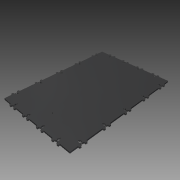
# Autodesk Inventor part: bottom
Saved by Autodesk Inventor 2014 (Build 180170000, 170)
## iProperties
Created: 2013-12-07
Part Number: bottom
Material: Plywood, Finish
Document SubType Name: Modeling
Designer: buben
Density: 0.552 g/cm^3
Appearance: Plywood - New
Author: buben
Subject: Laser Cutted
Autodesk Inventor part; units mm, degrees
ref_plane "YZ Plane" through (0, 0, 0) normal (1, 0, 0) x (0, 1, 0)
ref_plane "XZ Plane" through (0, 0, 0) normal (0, 1, 0) x (-1, 0, 0)
ref_plane "XY Plane" through (0, 0, 0) normal (0, 0, 1) x (1, 0, 0)
sketch "Sketch1" plane through (0, 0, 0) normal (0, 0, 1) x (1, 0, 0)
  line L0 (0, 0) -> (336, 0)
  line L1 (336, 0) -> (336, 489)
  line L2 (336, 489) -> (0, 489)
  line L3 (0, 489) -> (0, 0)
  dimension "d0" = 336
  dimension "d1" = 489
  constraints: 8 end point, 2 parallel, 1 horizontal, 1 perpendicular
  measures "d0" distance of L0.start L0.end
  measures "d1" distance of L2.end L0.start
extrude "Extrusion1" add sketch "Sketch1" along normal blind 6.5
sketch "Sketch6" plane through (0, 0, 6.5) normal (0, 0, 1) x (1, 0, 0)
  line L0 (0, 0) -> (336, 0) projected
  line L1 (336, 0) -> (336, 489) projected
  line L2 (336, 489) -> (0, 489) projected
  line L3 (0, 489) -> (0, 0) projected
  line L4 (54.75, 0) -> (59.25, 0)
  line L5 (59.25, 16.3) -> (54.75, 16.3)
  line L6 (61.75, 12.3) -> (61.75, 5)
  line L7 (52.25, 5) -> (52.25, 12.3)
  line L8 (54.75, 16.3) -> (54.75, 12.3)
  line L9 (54.75, 5) -> (54.75, 0)
  line L10 (59.25, 0) -> (59.25, 5)
  line L11 (59.25, 12.3) -> (59.25, 16.3)
  line L12 (61.75, 5) -> (59.25, 5)
  line L13 (54.75, 5) -> (52.25, 5)
  line L14 (52.25, 12.3) -> (54.75, 12.3)
  line L15 (59.25, 12.3) -> (61.75, 12.3)
  line L16 (128.75, 0) -> (133.25, 0)
  line L17 (133.25, 16.3) -> (128.75, 16.3)
  line L18 (135.75, 12.3) -> (135.75, 5)
  line L19 (126.25, 5) -> (126.25, 12.3)
  line L20 (128.75, 16.3) -> (128.75, 12.3)
  line L21 (128.75, 5) -> (128.75, 0)
  line L22 (133.25, 0) -> (133.25, 5)
  line L23 (133.25, 12.3) -> (133.25, 16.3)
  line L24 (135.75, 5) -> (133.25, 5)
  line L25 (128.75, 5) -> (126.25, 5)
  line L26 (126.25, 12.3) -> (128.75, 12.3)
  line L27 (133.25, 12.3) -> (135.75, 12.3)
  line L28 (202.75, 0) -> (207.25, 0)
  line L29 (207.25, 16.3) -> (202.75, 16.3)
  line L30 (209.75, 12.3) -> (209.75, 5)
  line L31 (200.25, 5) -> (200.25, 12.3)
  line L32 (202.75, 16.3) -> (202.75, 12.3)
  line L33 (202.75, 5) -> (202.75, 0)
  line L34 (207.25, 0) -> (207.25, 5)
  line L35 (207.25, 12.3) -> (207.25, 16.3)
  line L36 (209.75, 5) -> (207.25, 5)
  line L37 (202.75, 5) -> (200.25, 5)
  line L38 (200.25, 12.3) -> (202.75, 12.3)
  line L39 (207.25, 12.3) -> (209.75, 12.3)
  line L40 (276.75, 0) -> (281.25, 0)
  line L41 (281.25, 16.3) -> (276.75, 16.3)
  line L42 (283.75, 12.3) -> (283.75, 5)
  line L43 (274.25, 5) -> (274.25, 12.3)
  line L44 (276.75, 16.3) -> (276.75, 12.3)
  line L45 (276.75, 5) -> (276.75, 0)
  line L46 (281.25, 0) -> (281.25, 5)
  line L47 (281.25, 12.3) -> (281.25, 16.3)
  line L48 (283.75, 5) -> (281.25, 5)
  line L49 (276.75, 5) -> (274.25, 5)
  line L50 (274.25, 12.3) -> (276.75, 12.3)
  line L51 (281.25, 12.3) -> (283.75, 12.3)
  line L52 (0, 244.5) -> (336, 244.5) construction
  line L53 (54.75, 489) -> (59.25, 489)
  line L54 (59.25, 472.7) -> (54.75, 472.7)
  line L55 (61.75, 476.7) -> (61.75, 484)
  line L56 (52.25, 484) -> (52.25, 476.7)
  line L57 (54.75, 472.7) -> (54.75, 476.7)
  line L58 (54.75, 484) -> (54.75, 489)
  line L59 (59.25, 489) -> (59.25, 484)
  line L60 (59.25, 476.7) -> (59.25, 472.7)
  line L61 (61.75, 484) -> (59.25, 484)
  line L62 (54.75, 484) -> (52.25, 484)
  line L63 (52.25, 476.7) -> (54.75, 476.7)
  line L64 (59.25, 476.7) -> (61.75, 476.7)
  line L65 (128.75, 484) -> (126.25, 484)
  line L66 (135.75, 484) -> (133.25, 484)
  line L67 (128.75, 484) -> (128.75, 489)
  line L68 (128.75, 489) -> (133.25, 489)
  line L69 (133.25, 489) -> (133.25, 484)
  line L70 (126.25, 476.7) -> (128.75, 476.7)
  line L71 (126.25, 484) -> (126.25, 476.7)
  line L72 (133.25, 476.7) -> (135.75, 476.7)
  line L73 (135.75, 476.7) -> (135.75, 484)
  line L74 (128.75, 472.7) -> (128.75, 476.7)
  line L75 (133.25, 476.7) -> (133.25, 472.7)
  line L76 (133.25, 472.7) -> (128.75, 472.7)
  line L77 (202.75, 484) -> (200.25, 484)
  line L78 (209.75, 484) -> (207.25, 484)
  line L79 (202.75, 484) -> (202.75, 489)
  line L80 (202.75, 489) -> (207.25, 489)
  line L81 (207.25, 489) -> (207.25, 484)
  line L82 (200.25, 476.7) -> (202.75, 476.7)
  line L83 (200.25, 484) -> (200.25, 476.7)
  line L84 (207.25, 476.7) -> (209.75, 476.7)
  line L85 (209.75, 476.7) -> (209.75, 484)
  line L86 (202.75, 472.7) -> (202.75, 476.7)
  line L87 (207.25, 476.7) -> (207.25, 472.7)
  line L88 (207.25, 472.7) -> (202.75, 472.7)
  line L89 (276.75, 484) -> (274.25, 484)
  line L90 (283.75, 484) -> (281.25, 484)
  line L91 (276.75, 484) -> (276.75, 489)
  line L92 (276.75, 489) -> (281.25, 489)
  line L93 (281.25, 489) -> (281.25, 484)
  line L94 (274.25, 476.7) -> (276.75, 476.7)
  line L95 (274.25, 484) -> (274.25, 476.7)
  line L96 (281.25, 476.7) -> (283.75, 476.7)
  line L97 (283.75, 476.7) -> (283.75, 484)
  line L98 (276.75, 472.7) -> (276.75, 476.7)
  line L99 (281.25, 476.7) -> (281.25, 472.7)
  line L100 (281.25, 472.7) -> (276.75, 472.7)
  line L101 (16.3, 47.75) -> (16.3, 43.25)
  line L102 (0, 43.25) -> (0, 47.75)
  line L103 (5, 50.25) -> (12.3, 50.25)
  line L104 (12.3, 40.75) -> (5, 40.75)
  line L105 (5, 40.75) -> (5, 43.25)
  line L106 (5, 47.75) -> (5, 50.25)
  line L107 (12.3, 50.25) -> (12.3, 47.75)
  line L108 (12.3, 43.25) -> (12.3, 40.75)
  line L109 (0, 47.75) -> (5, 47.75)
  line L110 (12.3, 47.75) -> (16.3, 47.75)
  line L111 (16.3, 43.25) -> (12.3, 43.25)
  line L112 (5, 43.25) -> (0, 43.25)
  line L113 (168, 489) -> (168, 0) construction
  line L114 (16.3, 147.25) -> (16.3, 142.75)
  line L115 (0, 142.75) -> (0, 147.25)
  line L116 (5, 149.75) -> (12.3, 149.75)
  line L117 (12.3, 140.25) -> (5, 140.25)
  line L118 (5, 140.25) -> (5, 142.75)
  line L119 (5, 147.25) -> (5, 149.75)
  line L120 (12.3, 149.75) -> (12.3, 147.25)
  line L121 (12.3, 142.75) -> (12.3, 140.25)
  line L122 (0, 147.25) -> (5, 147.25)
  line L123 (12.3, 147.25) -> (16.3, 147.25)
  line L124 (16.3, 142.75) -> (12.3, 142.75)
  line L125 (5, 142.75) -> (0, 142.75)
  line L126 (16.3, 246.75) -> (16.3, 242.25)
  line L127 (0, 242.25) -> (0, 246.75)
  line L128 (5, 249.25) -> (12.3, 249.25)
  line L129 (12.3, 239.75) -> (5, 239.75)
  line L130 (5, 239.75) -> (5, 242.25)
  line L131 (5, 246.75) -> (5, 249.25)
  line L132 (12.3, 249.25) -> (12.3, 246.75)
  line L133 (12.3, 242.25) -> (12.3, 239.75)
  line L134 (0, 246.75) -> (5, 246.75)
  line L135 (12.3, 246.75) -> (16.3, 246.75)
  line L136 (16.3, 242.25) -> (12.3, 242.25)
  line L137 (5, 242.25) -> (0, 242.25)
  line L138 (16.3, 346.25) -> (16.3, 341.75)
  line L139 (0, 341.75) -> (0, 346.25)
  line L140 (5, 348.75) -> (12.3, 348.75)
  line L141 (12.3, 339.25) -> (5, 339.25)
  line L142 (5, 339.25) -> (5, 341.75)
  line L143 (5, 346.25) -> (5, 348.75)
  line L144 (12.3, 348.75) -> (12.3, 346.25)
  line L145 (12.3, 341.75) -> (12.3, 339.25)
  line L146 (0, 346.25) -> (5, 346.25)
  line L147 (12.3, 346.25) -> (16.3, 346.25)
  line L148 (16.3, 341.75) -> (12.3, 341.75)
  line L149 (5, 341.75) -> (0, 341.75)
  line L150 (16.3, 445.75) -> (16.3, 441.25)
  line L151 (0, 441.25) -> (0, 445.75)
  line L152 (5, 448.25) -> (12.3, 448.25)
  line L153 (12.3, 438.75) -> (5, 438.75)
  line L154 (5, 438.75) -> (5, 441.25)
  line L155 (5, 445.75) -> (5, 448.25)
  line L156 (12.3, 448.25) -> (12.3, 445.75)
  line L157 (12.3, 441.25) -> (12.3, 438.75)
  line L158 (0, 445.75) -> (5, 445.75)
  line L159 (12.3, 445.75) -> (16.3, 445.75)
  line L160 (16.3, 441.25) -> (12.3, 441.25)
  line L161 (5, 441.25) -> (0, 441.25)
  line L162 (319.7, 47.75) -> (319.7, 43.25)
  line L163 (336, 43.25) -> (336, 47.75)
  line L164 (331, 50.25) -> (323.7, 50.25)
  line L165 (323.7, 40.75) -> (331, 40.75)
  line L166 (331, 40.75) -> (331, 43.25)
  line L167 (331, 47.75) -> (331, 50.25)
  line L168 (323.7, 50.25) -> (323.7, 47.75)
  line L169 (323.7, 43.25) -> (323.7, 40.75)
  line L170 (336, 47.75) -> (331, 47.75)
  line L171 (323.7, 47.75) -> (319.7, 47.75)
  line L172 (319.7, 43.25) -> (323.7, 43.25)
  line L173 (331, 43.25) -> (336, 43.25)
  line L174 (323.7, 147.25) -> (319.7, 147.25)
  line L175 (319.7, 147.25) -> (319.7, 142.75)
  line L176 (319.7, 142.75) -> (323.7, 142.75)
  line L177 (323.7, 149.75) -> (323.7, 147.25)
  line L178 (323.7, 142.75) -> (323.7, 140.25)
  line L179 (323.7, 140.25) -> (331, 140.25)
  line L180 (331, 149.75) -> (323.7, 149.75)
  line L181 (331, 140.25) -> (331, 142.75)
  line L182 (331, 147.25) -> (331, 149.75)
  line L183 (336, 147.25) -> (331, 147.25)
  line L184 (336, 142.75) -> (336, 147.25)
  line L185 (331, 142.75) -> (336, 142.75)
  line L186 (323.7, 246.75) -> (319.7, 246.75)
  line L187 (319.7, 246.75) -> (319.7, 242.25)
  line L188 (319.7, 242.25) -> (323.7, 242.25)
  line L189 (323.7, 249.25) -> (323.7, 246.75)
  line L190 (323.7, 242.25) -> (323.7, 239.75)
  line L191 (323.7, 239.75) -> (331, 239.75)
  line L192 (331, 249.25) -> (323.7, 249.25)
  line L193 (331, 239.75) -> (331, 242.25)
  line L194 (331, 246.75) -> (331, 249.25)
  line L195 (336, 246.75) -> (331, 246.75)
  line L196 (336, 242.25) -> (336, 246.75)
  line L197 (331, 242.25) -> (336, 242.25)
  line L198 (323.7, 346.25) -> (319.7, 346.25)
  line L199 (319.7, 346.25) -> (319.7, 341.75)
  line L200 (319.7, 341.75) -> (323.7, 341.75)
  line L201 (323.7, 348.75) -> (323.7, 346.25)
  line L202 (323.7, 341.75) -> (323.7, 339.25)
  line L203 (323.7, 339.25) -> (331, 339.25)
  line L204 (331, 348.75) -> (323.7, 348.75)
  line L205 (331, 339.25) -> (331, 341.75)
  line L206 (331, 346.25) -> (331, 348.75)
  line L207 (336, 346.25) -> (331, 346.25)
  line L208 (336, 341.75) -> (336, 346.25)
  line L209 (331, 341.75) -> (336, 341.75)
  line L210 (323.7, 445.75) -> (319.7, 445.75)
  line L211 (319.7, 445.75) -> (319.7, 441.25)
  line L212 (319.7, 441.25) -> (323.7, 441.25)
  line L213 (323.7, 448.25) -> (323.7, 445.75)
  line L214 (323.7, 441.25) -> (323.7, 438.75)
  line L215 (323.7, 438.75) -> (331, 438.75)
  line L216 (331, 448.25) -> (323.7, 448.25)
  line L217 (331, 438.75) -> (331, 441.25)
  line L218 (331, 445.75) -> (331, 448.25)
  line L219 (336, 445.75) -> (331, 445.75)
  line L220 (336, 441.25) -> (336, 445.75)
  line L221 (331, 441.25) -> (336, 441.25)
  point P0 (57, 16.3)
  point P1 (131, 16.3)
  point P2 (205, 16.3)
  point P3 (279, 16.3)
  point P4 (57, 472.7)
  point P5 (131, 472.7)
  point P6 (205, 472.7)
  point P7 (279, 472.7)
  point P8 (16.3, 45.5)
  point P9 (16.3, 145)
  point P10 (16.3, 244.5)
  point P11 (16.3, 344)
  point P12 (16.3, 443.5)
  point P13 (319.7, 45.5)
  point P14 (319.7, 145)
  point P15 (319.7, 244.5)
  point P16 (319.7, 344)
  point P17 (319.7, 443.5)
  dimension "d66" = 4.5
  dimension "d67" = 7.3
  dimension "d68" = 5
  dimension "d69" = 4
  dimension "d70" = 2.5
  dimension "d71" = 2.5
  dimension "d72" = 57
  dimension "d75" = 74
  dimension "d80" = 4.5
  dimension "d81" = 7.3
  dimension "d82" = 5
  dimension "d83" = 4
  dimension "d84" = 2.5
  dimension "d85" = 2.5
  dimension "d86" = 45.5
  dimension "d89" = 99.5
  constraints: 436 end point, 117 symmetric about line, 20 parallel, 9 collinear, 8 perpendicular, 7 horizontal, 6 midpoint, 1 point on line, 1 vertical, 175 other
  measures "d66" distance of L5.start L5.end
  measures "d67" distance of L6.start L6.end
  measures "d68" distance of L4.end L10.end
  measures "d69" distance of L11.start L5.start
  measures "d70" distance of L7.end L8.end
  measures "d71" distance of L11.start L6.start
  measures "d72" distance from line of L3 point (57, 16.3)
  measures "d75" distance of L7.start L25.end
  measures "d80" distance of L101.start L101.end
  measures "d81" distance of L104.start L104.end
  measures "d82" distance of L105.end L102.start
  measures "d83" distance of L101.end L108.start
  measures "d84" distance of L104.end L105.end
  measures "d85" distance of L106.start L103.start
  measures "d86" distance from line of L0 point (16.3, 45.5)
  measures "d89" distance of L101.start L123.end
extrude "Extrusion6" cut sketch "Sketch6" against normal through all contours L9 L13 L7 L14 L8 L5 L11 L15 L6 L12 L10 L0 | L3 L109 L106 L103 L107 L110 L101 L111 L108 L104 L105 L112 | L21 L25 L19 L26 L20 L17 L23 L27 L18 L24 L22 L0 | L3 L122 L119 L116 L120 L123 L114 L124 L121 L117 L118 L125 | L33 L37 L31 L38 L32 L29 L35 L39 L30 L36 L34 L0 | L3 L134 L131 L128 L132 L135 L126 L136 L133 L129 L130 L137 | L45 L49 L43 L50 L44 L41 L47 L51 L42 L48 L46 L0 | L3 L146 L143 L140 L144 L147 L138 L148 L145 L141 L142 L149 | L3 L158 L155 L152 L156 L159 L150 L160 L157 L153 L154 L161 | L173 L166 L165 L169 L172 L162 L171 L168 L164 L167 L170 L1 | L185 L181 L179 L178 L176 L175 L174 L177 L180 L182 L183 L1 | L2 L59 L61 L55 L64 L60 L54 L57 L63 L56 L62 L58 | L197 L193 L191 L190 L188 L187 L186 L189 L192 L194 L195 L1 | L2 L69 L66 L73 L72 L75 L76 L74 L70 L71 L65 L67 | L209 L205 L203 L202 L200 L199 L198 L201 L204 L206 L207 L1 | L2 L81 L78 L85 L84 L87 L88 L86 L82 L83 L77 L79 | L221 L217 L215 L214 L212 L211 L210 L213 L216 L218 L219 L1 | L2 L93 L90 L97 L96 L99 L100 L98 L94 L95 L89 L91
sketch "Sketch7" plane through (0, 0, 6.5) normal (0, 0, 1) x (1, 0, 0)
  line L0 (319.7, 242.25) -> (319.7, 246.75) projected
  line L1 (202.75, 489) -> (133.25, 489) projected
  line L2 (16.3, 246.75) -> (16.3, 242.25) projected
  line L3 (0, 142.75) -> (0, 47.75) projected
  line L4 (16.3, 47.75) -> (16.3, 43.25) projected
  line L5 (0, 43.25) -> (0, 0) projected
  line L6 (0, 0) -> (54.75, 0) projected
  line L7 (54.75, 16.3) -> (59.25, 16.3) projected
  line L8 (59.25, 0) -> (128.75, 0) projected
  line L9 (133.25, 0) -> (202.75, 0) projected
  line L10 (41.5, 0) -> (49.5, 0)
  line L11 (49.5, 0) -> (49.5, -4.5)
  line L12 (47.5, -6.5) -> (43.5, -6.5)
  line L13 (41.5, -4.5) -> (41.5, 0)
  line L14 (64.5, 0) -> (72.5, 0)
  line L15 (72.5, 0) -> (72.5, -4.5)
  line L16 (70.5, -6.5) -> (66.5, -6.5)
  line L17 (64.5, -4.5) -> (64.5, 0)
  line L18 (0, 38) -> (-4.5, 38)
  line L19 (-6.5, 36) -> (-6.5, 32)
  line L20 (-4.5, 30) -> (0, 30)
  line L21 (0, 30) -> (0, 38)
  line L22 (0, 61) -> (-4.5, 61)
  line L23 (-6.5, 59) -> (-6.5, 55)
  line L24 (-4.5, 53) -> (0, 53)
  line L25 (0, 53) -> (0, 61)
  arc A0 (-6.5, 55) -> (-4.5, 53) centre (-4.5, 55) ccw
  arc A1 (-4.5, 61) -> (-6.5, 59) centre (-4.5, 59) ccw
  arc A2 (-4.5, 38) -> (-6.5, 36) centre (-4.5, 36) ccw
  arc A3 (-6.5, 32) -> (-4.5, 30) centre (-4.5, 32) ccw
  arc A4 (41.5, -4.5) -> (43.5, -6.5) centre (43.5, -4.5) ccw
  arc A5 (47.5, -6.5) -> (49.5, -4.5) centre (47.5, -4.5) ccw
  arc A6 (64.5, -4.5) -> (66.5, -6.5) centre (66.5, -4.5) ccw
  arc A7 (70.5, -6.5) -> (72.5, -4.5) centre (70.5, -4.5) ccw
  line L26 (168, 489) -> (168, 0) construction
  line L27 (115.5, 0) -> (123.5, 0)
  line L28 (123.5, 0) -> (123.5, -4.5)
  line L29 (121.5, -6.5) -> (117.5, -6.5)
  line L30 (115.5, -4.5) -> (115.5, 0)
  line L31 (138.5, 0) -> (146.5, 0)
  line L32 (146.5, 0) -> (146.5, -4.5)
  line L33 (144.5, -6.5) -> (140.5, -6.5)
  line L34 (138.5, -4.5) -> (138.5, 0)
  arc A8 (115.5, -4.5) -> (117.5, -6.5) centre (117.5, -4.5) ccw
  arc A9 (121.5, -6.5) -> (123.5, -4.5) centre (121.5, -4.5) ccw
  arc A10 (138.5, -4.5) -> (140.5, -6.5) centre (140.5, -4.5) ccw
  arc A11 (144.5, -6.5) -> (146.5, -4.5) centre (144.5, -4.5) ccw
  line L35 (189.5, 0) -> (197.5, 0)
  line L36 (197.5, 0) -> (197.5, -4.5)
  line L37 (195.5, -6.5) -> (191.5, -6.5)
  line L38 (189.5, -4.5) -> (189.5, 0)
  line L39 (212.5, 0) -> (220.5, 0)
  line L40 (220.5, 0) -> (220.5, -4.5)
  line L41 (218.5, -6.5) -> (214.5, -6.5)
  line L42 (212.5, -4.5) -> (212.5, 0)
  arc A12 (189.5, -4.5) -> (191.5, -6.5) centre (191.5, -4.5) ccw
  arc A13 (195.5, -6.5) -> (197.5, -4.5) centre (195.5, -4.5) ccw
  arc A14 (212.5, -4.5) -> (214.5, -6.5) centre (214.5, -4.5) ccw
  arc A15 (218.5, -6.5) -> (220.5, -4.5) centre (218.5, -4.5) ccw
  line L43 (263.5, 0) -> (271.5, 0)
  line L44 (271.5, 0) -> (271.5, -4.5)
  line L45 (269.5, -6.5) -> (265.5, -6.5)
  line L46 (263.5, -4.5) -> (263.5, 0)
  line L47 (286.5, 0) -> (294.5, 0)
  line L48 (294.5, 0) -> (294.5, -4.5)
  line L49 (292.5, -6.5) -> (288.5, -6.5)
  line L50 (286.5, -4.5) -> (286.5, 0)
  arc A16 (263.5, -4.5) -> (265.5, -6.5) centre (265.5, -4.5) ccw
  arc A17 (269.5, -6.5) -> (271.5, -4.5) centre (269.5, -4.5) ccw
  arc A18 (286.5, -4.5) -> (288.5, -6.5) centre (288.5, -4.5) ccw
  arc A19 (292.5, -6.5) -> (294.5, -4.5) centre (292.5, -4.5) ccw
  line L51 (0, 137.5) -> (-4.5, 137.5)
  line L52 (-6.5, 135.5) -> (-6.5, 131.5)
  line L53 (-4.5, 129.5) -> (0, 129.5)
  line L54 (0, 129.5) -> (0, 137.5)
  line L55 (0, 160.5) -> (-4.5, 160.5)
  line L56 (-6.5, 158.5) -> (-6.5, 154.5)
  line L57 (-4.5, 152.5) -> (0, 152.5)
  line L58 (0, 152.5) -> (0, 160.5)
  arc A20 (-6.5, 154.5) -> (-4.5, 152.5) centre (-4.5, 154.5) ccw
  arc A21 (-4.5, 160.5) -> (-6.5, 158.5) centre (-4.5, 158.5) ccw
  arc A22 (-4.5, 137.5) -> (-6.5, 135.5) centre (-4.5, 135.5) ccw
  arc A23 (-6.5, 131.5) -> (-4.5, 129.5) centre (-4.5, 131.5) ccw
  line L59 (0, 237) -> (-4.5, 237)
  line L60 (-6.5, 235) -> (-6.5, 231)
  line L61 (-4.5, 229) -> (0, 229)
  line L62 (0, 229) -> (0, 237)
  line L63 (0, 260) -> (-4.5, 260)
  line L64 (-6.5, 258) -> (-6.5, 254)
  line L65 (-4.5, 252) -> (0, 252)
  line L66 (0, 252) -> (0, 260)
  arc A24 (-6.5, 254) -> (-4.5, 252) centre (-4.5, 254) ccw
  arc A25 (-4.5, 260) -> (-6.5, 258) centre (-4.5, 258) ccw
  arc A26 (-4.5, 237) -> (-6.5, 235) centre (-4.5, 235) ccw
  arc A27 (-6.5, 231) -> (-4.5, 229) centre (-4.5, 231) ccw
  line L67 (0, 336.5) -> (-4.5, 336.5)
  line L68 (-6.5, 334.5) -> (-6.5, 330.5)
  line L69 (-4.5, 328.5) -> (0, 328.5)
  line L70 (0, 328.5) -> (0, 336.5)
  line L71 (0, 359.5) -> (-4.5, 359.5)
  line L72 (-6.5, 357.5) -> (-6.5, 353.5)
  line L73 (-4.5, 351.5) -> (0, 351.5)
  line L74 (0, 351.5) -> (0, 359.5)
  arc A28 (-6.5, 353.5) -> (-4.5, 351.5) centre (-4.5, 353.5) ccw
  arc A29 (-4.5, 359.5) -> (-6.5, 357.5) centre (-4.5, 357.5) ccw
  arc A30 (-4.5, 336.5) -> (-6.5, 334.5) centre (-4.5, 334.5) ccw
  arc A31 (-6.5, 330.5) -> (-4.5, 328.5) centre (-4.5, 330.5) ccw
  line L75 (0, 436) -> (-4.5, 436)
  line L76 (-6.5, 434) -> (-6.5, 430)
  line L77 (-4.5, 428) -> (0, 428)
  line L78 (0, 428) -> (0, 436)
  line L79 (0, 459) -> (-4.5, 459)
  line L80 (-6.5, 457) -> (-6.5, 453)
  line L81 (-4.5, 451) -> (0, 451)
  line L82 (0, 451) -> (0, 459)
  arc A32 (-6.5, 453) -> (-4.5, 451) centre (-4.5, 453) ccw
  arc A33 (-4.5, 459) -> (-6.5, 457) centre (-4.5, 457) ccw
  arc A34 (-4.5, 436) -> (-6.5, 434) centre (-4.5, 434) ccw
  arc A35 (-6.5, 430) -> (-4.5, 428) centre (-4.5, 430) ccw
  line L83 (336, 38) -> (340.5, 38)
  line L84 (342.5, 36) -> (342.5, 32)
  line L85 (340.5, 30) -> (336, 30)
  line L86 (336, 30) -> (336, 38)
  line L87 (336, 61) -> (340.5, 61)
  line L88 (342.5, 59) -> (342.5, 55)
  line L89 (340.5, 53) -> (336, 53)
  line L90 (336, 53) -> (336, 61)
  arc A36 (340.5, 53) -> (342.5, 55) centre (340.5, 55) ccw
  arc A37 (342.5, 59) -> (340.5, 61) centre (340.5, 59) ccw
  arc A38 (342.5, 36) -> (340.5, 38) centre (340.5, 36) ccw
  arc A39 (340.5, 30) -> (342.5, 32) centre (340.5, 32) ccw
  line L91 (340.5, 152.5) -> (336, 152.5)
  line L92 (336, 160.5) -> (340.5, 160.5)
  line L93 (336, 152.5) -> (336, 160.5)
  arc A40 (342.5, 158.5) -> (340.5, 160.5) centre (340.5, 158.5) ccw
  line L94 (342.5, 158.5) -> (342.5, 154.5)
  arc A41 (340.5, 152.5) -> (342.5, 154.5) centre (340.5, 154.5) ccw
  arc A42 (342.5, 135.5) -> (340.5, 137.5) centre (340.5, 135.5) ccw
  line L95 (342.5, 135.5) -> (342.5, 131.5)
  arc A43 (340.5, 129.5) -> (342.5, 131.5) centre (340.5, 131.5) ccw
  line L96 (336, 137.5) -> (340.5, 137.5)
  line L97 (340.5, 129.5) -> (336, 129.5)
  line L98 (336, 129.5) -> (336, 137.5)
  line L99 (340.5, 252) -> (336, 252)
  line L100 (336, 260) -> (340.5, 260)
  line L101 (336, 252) -> (336, 260)
  arc A44 (342.5, 258) -> (340.5, 260) centre (340.5, 258) ccw
  line L102 (342.5, 258) -> (342.5, 254)
  arc A45 (340.5, 252) -> (342.5, 254) centre (340.5, 254) ccw
  arc A46 (342.5, 235) -> (340.5, 237) centre (340.5, 235) ccw
  line L103 (342.5, 235) -> (342.5, 231)
  arc A47 (340.5, 229) -> (342.5, 231) centre (340.5, 231) ccw
  line L104 (336, 237) -> (340.5, 237)
  line L105 (340.5, 229) -> (336, 229)
  line L106 (336, 229) -> (336, 237)
  line L107 (340.5, 351.5) -> (336, 351.5)
  line L108 (336, 359.5) -> (340.5, 359.5)
  line L109 (336, 351.5) -> (336, 359.5)
  arc A48 (342.5, 357.5) -> (340.5, 359.5) centre (340.5, 357.5) ccw
  line L110 (342.5, 357.5) -> (342.5, 353.5)
  arc A49 (340.5, 351.5) -> (342.5, 353.5) centre (340.5, 353.5) ccw
  arc A50 (342.5, 334.5) -> (340.5, 336.5) centre (340.5, 334.5) ccw
  line L111 (342.5, 334.5) -> (342.5, 330.5)
  arc A51 (340.5, 328.5) -> (342.5, 330.5) centre (340.5, 330.5) ccw
  line L112 (336, 336.5) -> (340.5, 336.5)
  line L113 (340.5, 328.5) -> (336, 328.5)
  line L114 (336, 328.5) -> (336, 336.5)
  line L115 (340.5, 451) -> (336, 451)
  line L116 (336, 459) -> (340.5, 459)
  line L117 (336, 451) -> (336, 459)
  arc A52 (342.5, 457) -> (340.5, 459) centre (340.5, 457) ccw
  line L118 (342.5, 457) -> (342.5, 453)
  arc A53 (340.5, 451) -> (342.5, 453) centre (340.5, 453) ccw
  arc A54 (342.5, 434) -> (340.5, 436) centre (340.5, 434) ccw
  line L119 (342.5, 434) -> (342.5, 430)
  arc A55 (340.5, 428) -> (342.5, 430) centre (340.5, 430) ccw
  line L120 (336, 436) -> (340.5, 436)
  line L121 (340.5, 428) -> (336, 428)
  line L122 (336, 428) -> (336, 436)
  line L123 (16.3, 244.5) -> (319.7, 244.5) construction
  line L124 (41.5, 489) -> (49.5, 489)
  line L125 (49.5, 489) -> (49.5, 493.5)
  line L126 (47.5, 495.5) -> (43.5, 495.5)
  line L127 (41.5, 493.5) -> (41.5, 489)
  line L128 (64.5, 489) -> (72.5, 489)
  line L129 (72.5, 489) -> (72.5, 493.5)
  line L130 (70.5, 495.5) -> (66.5, 495.5)
  line L131 (64.5, 493.5) -> (64.5, 489)
  arc A56 (43.5, 495.5) -> (41.5, 493.5) centre (43.5, 493.5) ccw
  arc A57 (49.5, 493.5) -> (47.5, 495.5) centre (47.5, 493.5) ccw
  arc A58 (66.5, 495.5) -> (64.5, 493.5) centre (66.5, 493.5) ccw
  arc A59 (72.5, 493.5) -> (70.5, 495.5) centre (70.5, 493.5) ccw
  line L132 (123.5, 489) -> (123.5, 493.5)
  arc A60 (123.5, 493.5) -> (121.5, 495.5) centre (121.5, 493.5) ccw
  line L133 (121.5, 495.5) -> (117.5, 495.5)
  arc A61 (117.5, 495.5) -> (115.5, 493.5) centre (117.5, 493.5) ccw
  line L134 (115.5, 489) -> (123.5, 489)
  line L135 (115.5, 493.5) -> (115.5, 489)
  line L136 (138.5, 493.5) -> (138.5, 489)
  arc A62 (140.5, 495.5) -> (138.5, 493.5) centre (140.5, 493.5) ccw
  line L137 (144.5, 495.5) -> (140.5, 495.5)
  line L138 (146.5, 489) -> (146.5, 493.5)
  arc A63 (146.5, 493.5) -> (144.5, 495.5) centre (144.5, 493.5) ccw
  line L139 (138.5, 489) -> (146.5, 489)
  line L140 (197.5, 489) -> (197.5, 493.5)
  arc A64 (197.5, 493.5) -> (195.5, 495.5) centre (195.5, 493.5) ccw
  line L141 (195.5, 495.5) -> (191.5, 495.5)
  arc A65 (191.5, 495.5) -> (189.5, 493.5) centre (191.5, 493.5) ccw
  line L142 (189.5, 489) -> (197.5, 489)
  line L143 (189.5, 493.5) -> (189.5, 489)
  line L144 (212.5, 493.5) -> (212.5, 489)
  arc A66 (214.5, 495.5) -> (212.5, 493.5) centre (214.5, 493.5) ccw
  line L145 (218.5, 495.5) -> (214.5, 495.5)
  line L146 (220.5, 489) -> (220.5, 493.5)
  arc A67 (220.5, 493.5) -> (218.5, 495.5) centre (218.5, 493.5) ccw
  line L147 (212.5, 489) -> (220.5, 489)
  line L148 (271.5, 489) -> (271.5, 493.5)
  arc A68 (271.5, 493.5) -> (269.5, 495.5) centre (269.5, 493.5) ccw
  line L149 (269.5, 495.5) -> (265.5, 495.5)
  arc A69 (265.5, 495.5) -> (263.5, 493.5) centre (265.5, 493.5) ccw
  line L150 (263.5, 489) -> (271.5, 489)
  line L151 (263.5, 493.5) -> (263.5, 489)
  line L152 (286.5, 493.5) -> (286.5, 489)
  arc A70 (288.5, 495.5) -> (286.5, 493.5) centre (288.5, 493.5) ccw
  line L153 (292.5, 495.5) -> (288.5, 495.5)
  line L154 (294.5, 489) -> (294.5, 493.5)
  arc A71 (294.5, 493.5) -> (292.5, 495.5) centre (292.5, 493.5) ccw
  line L155 (286.5, 489) -> (294.5, 489)
  point P0 (16.3, 45.5)
  point P1 (57, 16.3)
  dimension "d96" = 2
  dimension "d97" = 8
  dimension "d98" = 8
  dimension "d99" = 8
  dimension "d100" = 8
  dimension "d101" = 6.5
  dimension "d102" = 6.5
  dimension "d103" = 15
  dimension "d104" = 15
  dimension "d105" = 7.5
  dimension "d106" = 7.5
  dimension "d109" = 74
  dimension "d116" = 99.5
  constraints: 292 end point, 144 point on circle, 144 symmetric about line, 72 centre point, 16 tangent, 8 parallel, 7 equal radius, 6 midpoint, 5 horizontal, 4 perpendicular, 4 point on line, 2 collinear, 1 vertical, 232 other
  measures "d96" radius of A0
  measures "d97" distance between parallel lines of L24 L22
  measures "d98" distance between parallel lines of L20 L18
  measures "d99" distance between parallel lines of L11 L13
  measures "d100" distance between parallel lines of L15 L17
  measures "d101" distance between parallel lines of L3 L23
  measures "d102" distance between parallel lines of L6 L12
  measures "d103" distance between parallel lines of L18 L24
  measures "d104" distance between parallel lines of L17 L11
  measures "d105" distance from line of point (16.3, 45.5) L18
  measures "d106" distance from line of point (57, 16.3) L11
  measures "d109" distance of L10.end L28.start
  measures "d116" distance of L24.end L57.end
extrude "Extrusion7" add sketch "Sketch7" against normal blind 6.5
sketch "Sketch8" plane through (0, 0, 6.5) normal (0, 0, 1) x (1, 0, 0)
  line L0 (0, 129.5) -> (0, 61) projected
  line L1 (146.5, 0) -> (189.5, 0) projected
  circle A0 centre (176.5, 67.3) radius 2.25
  dimension "d123" = 4.5
  dimension "d124" = 67.3
  dimension "d125" = 176.5
  constraints: 1 centre point
  measures "d123" diameter of A0
  measures "d124" distance from line of L1 A0.centre
  measures "d125" distance from line of L0 A0.centre
extrude "Extrusion8" cut sketch "Sketch8" against normal through all
body "Solid1"
